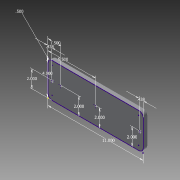
# Autodesk Inventor part: BasePlateDE
Saved by Autodesk Inventor 2015 (Build 190159000, 159)
## iProperties
Created: 2017-12-14
Part Number: BasePlateDE
Material: Generic
Document SubType Name: Modeling
Designer: Administrator
Density: 1 g/cm^3
Appearance: Default
Author: Administrator
Autodesk Inventor part; units mm, degrees
ref_plane "YZ Plane" through (0, 0, 0) normal (1, 0, 0) x (0, 1, 0)
ref_plane "XZ Plane" through (0, 0, 0) normal (0, 1, 0) x (-1, 0, 0)
ref_plane "XY Plane" through (0, 0, 0) normal (0, 0, 1) x (1, 0, 0)
sketch "Sketch1" plane through (0, 0, 0) normal (0, 0, 1) x (1, 0, 0)
  line L0 (12.7, 0) -> (266.7, 0)
  line L1 (279.4, 12.7) -> (279.4, 88.9)
  line L2 (266.7, 101.6) -> (12.7, 101.6)
  line L3 (0, 88.9) -> (0, 12.7)
  arc A0 (12.7, 101.6) -> (0, 88.9) centre (12.7, 88.9) ccw
  arc A1 (279.4, 88.9) -> (266.7, 101.6) centre (266.7, 88.9) ccw
  arc A2 (266.7, 0) -> (279.4, 12.7) centre (266.7, 12.7) ccw
  arc A3 (0, 12.7) -> (12.7, 0) centre (12.7, 12.7) ccw
  point P0 (0, 0)
  point P1 (279.4, 0)
  point P2 (0, 101.6)
  point P3 (11.1125, 50.8)
  point P4 (38.1, 50.8)
  point P5 (139.7, 50.8)
  point P6 (268.2875, 50.8)
  dimension "d0" = 101.6
  dimension "d1" = 279.4
  dimension "d2" = 12.7
  dimension "d5" = 11.1125
  dimension "d6" = 50.8
  dimension "d7" = 50.8
  dimension "d8" = 50.8
  dimension "d9" = 50.8
  dimension "d10" = 38.1
  dimension "d11" = 139.7
  dimension "d12" = 11.1125
  constraints: 8 end point, 8 point on circle, 8 tangent, 6 point on line, 4 centre point, 3 equal radius, 2 parallel, 1 horizontal, 1 perpendicular
  measures "d0" distance of point (0, 101.6) point (0, 0)
  measures "d1" distance of point (0, 0) point (279.4, 0)
  measures "d2" radius of A0
  measures "d5" distance from line of point (11.112, 50.8) L3
  measures "d6" distance from line of L0 point (11.112, 50.8)
  measures "d7" distance from line of L0 point (38.1, 50.8)
  measures "d8" distance from line of L0 point (139.7, 50.8)
  measures "d9" distance from line of L0 point (268.288, 50.8)
  measures "d10" distance from line of L3 point (38.1, 50.8)
  measures "d11" distance from line of L3 point (139.7, 50.8)
  measures "d12" distance from line of L1 point (268.288, 50.8)
extrude "Extrusion1" add sketch "Sketch1" against normal blind 12.7
hole "Hole1" at (11.1125, 50.8, 0) direction (0, 0, -1) diameter 6.35 end through all countersink diameter 12.7 countersink angle 82
hole "Hole2" at (268.2875, 50.8, 0) direction (0, 0, -1) diameter 6.35 end through all countersink diameter 12.7 countersink angle 82
hole "Hole3" at (38.1, 50.8, 0) direction (0, 0, -1) diameter 7.9375 end through all
hole "Hole4" at (139.7, 50.8, 0) direction (0, 0, -1) diameter 7.9375 end through all
chamfer "Chamfer1" distance 0.7937 angle 45 8 edges at (139.7, 101.6, 0) (275.6803, 97.8803, 0) (279.4, 50.8, 0) (275.6803, 3.7197, 0) (139.7, 0, 0) (3.7197, 3.7197, 0) (0, 50.8, 0) (3.7197, 97.8803, 0)
chamfer "Chamfer2" distance 0.7937 angle 45 8 edges at (139.7, 101.6, -12.7) (275.6803, 97.8803, -12.7) (279.4, 50.8, -12.7) (275.6803, 3.7197, -12.7) (139.7, 0, -12.7) (3.7197, 3.7197, -12.7) (0, 50.8, -12.7) (3.7197, 97.8803, -12.7)
sketch "Sketch2" plane through (0, 0, -12.7) normal (0, 0, -1) x (-1, 0, 0)
  point P0 (0, 0)
  point P1 (-266.7, 88.9)
  point P2 (-266.7, 12.7)
  point P3 (-12.7, 12.7)
  point P4 (-12.7, 88.9)
hole "Hole5" at (266.7, 88.9, -12.7) at (266.7, 12.7, -12.7) at (12.7, 12.7, -12.7) at (12.7, 88.9, -12.7) direction (0, 0, 1) diameter 3.302 depth 7.3025 thread size "8-32 UNC" class "2B" standard "ANSI Unified Screw Threads"
body "Solid1"
